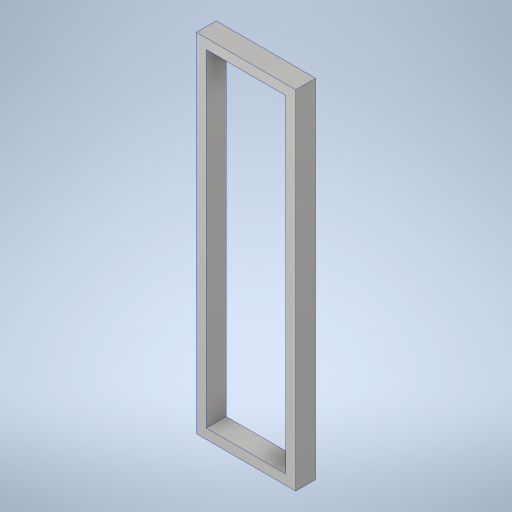
# Autodesk Inventor part: EL1-005
Saved by Autodesk Inventor 2023.4 (Build 274418000, 418)
## iProperties
Created: 2025-01-09
Part Number: EL1-005
Material: Aluminum 6061
Document SubType Name: Modeling
Designer: mavericks
Density: 2.7 g/cm^3
Appearance: Aluminum - Flat
Author: mavericks
Autodesk Inventor part; units mm, degrees
ref_plane "YZ Plane" through (0, 0, 0) normal (1, 0, 0) x (0, 1, 0)
ref_plane "XZ Plane" through (0, 0, 0) normal (0, 1, 0) x (-1, 0, 0)
ref_plane "XY Plane" through (0, 0, 0) normal (0, 0, 1) x (1, 0, 0)
sketch "Sketch1" plane through (0, 0, 0) normal (0, 0, 1) x (1, 0, 0)
  line L0 (-127, 444.5) -> (127, 444.5)
  line L1 (127, 444.5) -> (127, -444.5)
  line L2 (127, -444.5) -> (-127, -444.5)
  line L3 (-127, -444.5) -> (-127, 444.5)
  line L4 (-127, 444.5) -> (127, -444.5) construction
  line L5 (127, 444.5) -> (-127, -444.5) construction
  line L6 (-101.6, 419.1) -> (101.6, 419.1)
  line L7 (101.6, 419.1) -> (101.6, -419.1)
  line L8 (101.6, -419.1) -> (-101.6, -419.1)
  line L9 (-101.6, -419.1) -> (-101.6, 419.1)
  point P0 (0, 0)
  dimension "d0" = 254
  dimension "d1" = 889
  dimension "d4" = 25.4
  constraints: 20 end point, 4 parallel, 2 midpoint, 2 perpendicular, 1 horizontal, 3 other
  measures "d0" distance of L1.end L2.end
  measures "d1" distance of L0.end L1.end
  measures "d4" distance between parallel lines of L3 L9
extrude "Extrusion1" add sketch "Sketch1" along normal blind 50.8
body "Solid1"
